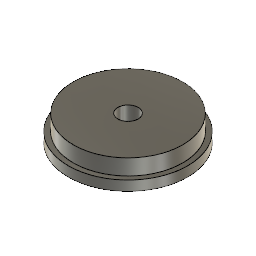
4-Roller_End_Cap v2 (Autodesk Fusion 360 design; units mm, degrees)
Autodesk Fusion 360 part; units mm, degrees
sketch "Roller_End_Cap_Outter" plane through (0, 0, 0) normal (0, 0, 1) x (1, 0, 0)
  circle A0 centre (0, 0) radius 381
  dimension "d2" = 762
  measures "d2" diameter of A0
extrude "Extrude1" add sketch "Roller_End_Cap_Outter" along normal blind 63.5
sketch "Roller_End_Cap_Inner" plane through (0, 0, 63.5) normal (0, 0, 1) x (-1, 0, 0)
  circle A0 centre (0, 0) radius 381
  circle A1 centre (0, 0) radius 349.25
  dimension "d7" = 698.5
  measures "d7" diameter of A1
extrude "Extrude3" add sketch "Roller_End_Cap_Inner" along normal blind 100 contours A1
sketch "Shaft Hole" plane through (0, 0, 163.5) normal (0, 0, 1) x (-1, 0, 0)
  circle A0 centre (0, 0) radius 349.25
  circle A1 centre (0, 0) radius 64.5
  dimension "d10" = 129
  measures "d10" diameter of A1
extrude "Extrude4" cut sketch "Shaft Hole" against normal through all contours A1
named bodies: "Roller_End_Cap"
